Autodesk Fusion 360 part; units mm, degrees
note: some values were not read from the file. Set by a fixed rule: which face or edge a step refers to.
(part 3 of 5)
sketch "Sketch19" plane through (0, 5, 0) normal (0, 1, 0) x (-1, 0, 0)
  line L0 (-11.62, 44.17) -> (-67.5, 44.17) construction
  line L1 (-115.5, 44.17) -> (-115.5, -27.83) construction
  line L2 (-115.5, -27.83) -> (-120.5, -27.83) construction
  line L3 (-120.5, -27.83) -> (-120.5, -39.83) construction
  line L4 (-120.5, -39.83) -> (67.5, -39.83) construction
  line L5 (-72.5, 2.17) -> (-115.5, 2.17) construction
  circle A0 centre (-94, 2.17) radius 1.5
  circle A1 centre (-109, -33.83) radius 1.5
  circle A2 centre (-101.5, -33.83) radius 1.5
  circle A3 centre (-94, -33.83) radius 1.5
  circle A4 centre (-86.5, -33.83) radius 1.5
  circle A5 centre (-79, -33.83) radius 1.5
  circle A6 centre (-109, -21.83) radius 1.5
  circle A7 centre (-101.5, -21.83) radius 1.5
  circle A8 centre (-94, -21.83) radius 1.5
  circle A9 centre (-86.5, -21.83) radius 1.5
  circle A10 centre (-79, -21.83) radius 1.5
  circle A11 centre (-109, -9.83) radius 1.5
  circle A12 centre (-101.5, -9.83) radius 1.5
  circle A13 centre (-94, -9.83) radius 1.5
  circle A14 centre (-86.5, -9.83) radius 1.5
  circle A15 centre (-79, -9.83) radius 1.5
  circle A16 centre (-109, 2.17) radius 1.5
  circle A17 centre (-101.5, 2.17) radius 1.5
  circle A18 centre (-86.5, 2.17) radius 1.5
  circle A19 centre (-79, 2.17) radius 1.5
  circle A20 centre (-109, 14.17) radius 1.5
  circle A21 centre (-101.5, 14.17) radius 1.5
  circle A22 centre (-94, 14.17) radius 1.5
  circle A23 centre (-86.5, 14.17) radius 1.5
  circle A24 centre (-79, 14.17) radius 1.5
  circle A25 centre (-109, 26.17) radius 1.5
  circle A26 centre (-101.5, 26.17) radius 1.5
  circle A27 centre (-94, 26.17) radius 1.5
  circle A28 centre (-86.5, 26.17) radius 1.5
  circle A29 centre (-79, 26.17) radius 1.5
  circle A30 centre (-109, 38.17) radius 1.5
  circle A31 centre (-101.5, 38.17) radius 1.5
  circle A32 centre (-94, 38.17) radius 1.5
  circle A33 centre (-86.5, 38.17) radius 1.5
  circle A34 centre (-79, 38.17) radius 1.5
  line L6 (-79, -33.83) -> (-79, -21.83) construction
  line L7 (-79, -21.83) -> (-86.5, -21.83) construction
  line L8 (-86.5, -21.83) -> (-86.5, -33.83) construction
  line L9 (-86.5, -33.83) -> (-79, -33.83) construction
  line L10 (-79, -27.83) -> (-86.5, -27.83) construction
  line L11 (-82.75, -33.83) -> (-82.75, -21.83) construction
  circle A35 centre (-82.75, -27.83) radius 1.5
  circle A36 centre (-90.25, -27.83) radius 1.5
  circle A37 centre (-97.75, -27.83) radius 1.5
  circle A38 centre (-105.25, -27.83) radius 1.5
  circle A39 centre (-82.75, -15.83) radius 1.5
  circle A40 centre (-90.25, -15.83) radius 1.5
  circle A41 centre (-97.75, -15.83) radius 1.5
  circle A42 centre (-105.25, -15.83) radius 1.5
  circle A43 centre (-82.75, -3.83) radius 1.5
  circle A44 centre (-90.25, -3.83) radius 1.5
  circle A45 centre (-97.75, -3.83) radius 1.5
  circle A46 centre (-105.25, -3.83) radius 1.5
  circle A47 centre (-82.75, 8.17) radius 1.5
  circle A48 centre (-90.25, 8.17) radius 1.5
  circle A49 centre (-97.75, 8.17) radius 1.5
  circle A50 centre (-105.25, 8.17) radius 1.5
  circle A51 centre (-82.75, 20.17) radius 1.5
  circle A52 centre (-90.25, 20.17) radius 1.5
  circle A53 centre (-97.75, 20.17) radius 1.5
  circle A54 centre (-105.25, 20.17) radius 1.5
  circle A55 centre (-82.75, 32.17) radius 1.5
  circle A56 centre (-90.25, 32.17) radius 1.5
  circle A57 centre (-97.75, 32.17) radius 1.5
  circle A58 centre (-105.25, 32.17) radius 1.5
  circle A59 centre (-31.75, 6.0325) radius 1.5
  circle A60 centre (-31.75, -18.0975) radius 1.5
  circle A61 centre (-6.35, -18.0975) radius 1.5
  circle A62 centre (-6.35, 18.0975) radius 1.5
  circle A63 centre (19.05, 18.0975) radius 1.5
  circle A64 centre (6.35, -18.0975) radius 1.5
  circle A65 centre (31.75, 6.0325) radius 1.5
  circle A66 centre (44.45, -6.0325) radius 1.5
  circle A67 centre (38.1, 24.13) radius 1.5
  circle A68 centre (0, 24.13) radius 1.5
  circle A69 centre (-25.4, -24.13) radius 1.5
  circle A70 centre (-12.7, -24.13) radius 1.5
  circle A71 centre (12.7, 12.065) radius 1.5
  circle A72 centre (50.8, -24.13) radius 1.5
  circle A73 centre (-50.8, -24.13) radius 1.5
  circle A74 centre (12.7, -12.065) radius 1.5
  circle A75 centre (-25.4, -12.065) radius 1.5
  circle A76 centre (50.8, 12.065) radius 1.5
  circle A77 centre (-38.1, 0) radius 1.5
  circle A78 centre (-50.8, 24.13) radius 1.5
  circle A79 centre (-12.7, -12.065) radius 1.5
  circle A80 centre (-38.1, -12.065) radius 1.5
  circle A81 centre (-38.1, -24.13) radius 1.5
  circle A82 centre (25.4, 0) radius 1.5
  circle A83 centre (25.4, -24.13) radius 1.5
  circle A84 centre (12.7, -24.13) radius 1.5
  circle A85 centre (38.1, -12.065) radius 1.5
  circle A86 centre (-38.1, 24.13) radius 1.5
  circle A87 centre (0, 12.065) radius 1.5
  circle A88 centre (-25.4, 0) radius 1.5
  circle A89 centre (44.45, -18.0975) radius 1.5
  circle A90 centre (31.75, 18.0975) radius 1.5
  circle A91 centre (19.05, -18.0975) radius 1.5
  circle A92 centre (19.05, 6.0325) radius 1.5
  circle A93 centre (-6.35, 6.0325) radius 1.5
  circle A94 centre (-6.35, -6.0325) radius 1.5
  circle A95 centre (-31.75, -6.0325) radius 1.5
  circle A96 centre (-44.45, 6.0325) radius 1.5
  circle A97 centre (-31.75, 18.0975) radius 1.5
  circle A98 centre (-44.45, -18.0975) radius 1.5
  circle A99 centre (-19.05, -18.0975) radius 1.5
  circle A100 centre (-19.05, 18.0975) radius 1.5
  circle A101 centre (6.35, 18.0975) radius 1.5
  circle A102 centre (6.35, -6.0325) radius 1.5
  circle A103 centre (31.75, -6.0325) radius 1.5
  circle A104 centre (44.45, 6.0325) radius 1.5
  circle A105 centre (25.4, 24.13) radius 1.5
  circle A106 centre (38.1, 0) radius 1.5
  circle A107 centre (-50.8, -12.065) radius 1.5
  circle A108 centre (-25.4, 24.13) radius 1.5
  circle A109 centre (-38.1, 12.065) radius 1.5
  circle A110 centre (38.1, -24.13) radius 1.5
  circle A111 centre (-50.8, 0) radius 1.5
  circle A112 centre (50.8, -12.065) radius 1.5
  circle A113 centre (38.1, 12.065) radius 1.5
  circle A114 centre (-50.8, 12.065) radius 1.5
  circle A115 centre (0, -24.13) radius 1.5
  circle A116 centre (-12.7, 0) radius 1.5
  circle A117 centre (12.7, 24.13) radius 1.5
  circle A118 centre (25.4, 12.065) radius 1.5
  circle A119 centre (-25.4, 12.065) radius 1.5
  circle A120 centre (12.7, 0) radius 1.5
  circle A121 centre (-12.7, 24.13) radius 1.5
  circle A122 centre (25.4, -12.065) radius 1.5
  circle A123 centre (0, 0) radius 1.5
  circle A124 centre (50.8, 0) radius 1.5
  circle A125 centre (50.8, 24.13) radius 1.5
  circle A126 centre (0, -12.065) radius 1.5
  circle A127 centre (-12.7, 12.065) radius 1.5
  circle A128 centre (44.45, 18.0975) radius 1.5
  circle A129 centre (31.75, -18.0975) radius 1.5
  circle A130 centre (19.05, -6.0325) radius 1.5
  circle A131 centre (6.35, 6.0325) radius 1.5
  circle A132 centre (-19.05, 6.0325) radius 1.5
  circle A133 centre (-19.05, -6.0325) radius 1.5
  circle A134 centre (-44.45, -6.0325) radius 1.5
  circle A135 centre (-44.45, 18.0975) radius 1.5
  circle A136 centre (58.42, -31.75) radius 3.9
  circle A137 centre (58.42, 31.75) radius 3.9
  line L12 (67.5, 39.83) -> (-11.62, 39.83)
  line L13 (-11.62, 39.83) -> (-11.62, 44.17)
  line L14 (67.5, -39.83) -> (67.5, 39.83)
  circle A138 centre (-58.42, 31.75) radius 3.9
  circle A139 centre (-58.42, -31.75) radius 3.9
  line L15 (-67.5, 44.17) -> (-67.5, -22.83)
  line L16 (-67.5, -22.83) -> (-72.5, -22.83)
  line L17 (-72.5, -22.83) -> (-72.5, 44.17)
  line L18 (-72.5, 44.17) -> (-115.5, 44.17)
  line L19 (-94, 44.17) -> (-94, -39.83) construction
  line L20 (-72.5, 44.17) -> (-72.5, -39.83) construction
  dimension "d176" = 3
  dimension "d179" = 15
  dimension "d180" = 36
  dimension "d181" = 3
  dimension "d184" = -22.5
  dimension "d185" = 60
  constraint coincident L1 L5.end
  constraint perpendicular L1 L5
  constraint coincident A5.centre L6.start
  constraint coincident A10.centre L6.end
  constraint coincident A9.centre L7.end
  constraint coincident A4.centre L8.end
  constraint midpoint L6 L10.start
  constraint midpoint L8 L10.end
  constraint midpoint L9 L11.start
  constraint midpoint L7 L11.end
  constraint midpoint L10 A35.centre
  constraint midpoint L18 L19.start
  constraint coincident L4 L19.end
  constraint vertical L19
  constraint coincident L5 A0.centre
  constraint coincident A0.centre L19
  constraint coincident L17.end L18.start
  constraint coincident L4 L20.end
  constraint perpendicular L4 L20
  constraint midpoint L5.start L20
  measures "d176" diameter of A0
  measures "d181" diameter of A35
extrude "Extrude22" cut sketch "Sketch19" against normal up to surface (5 mm away) contours A0 | A1 | A2 | A3 | A4 | A5 | A6 | A7 | A8 | A9 | A10 | A11 | A12 | A13 | A14 | A15 | A16 | A17 | A18 | A19 | A20 | A21 | A22 | A23 | A24 | A25 | A26 | A27 | A28 | A29 | A30 | A31 | A32 | A33 | A34 | A35 | A36 | A37 | A38 | A39 | A40 | A41 | A42 | A43 | A44 | A45 | A46 | A47 | A48 | A49 | A50 | A51 | A52 | A53 | A54 | A55 | A56 | A57 | A58 bodies 1
fillet "Fillet2" [suppressed]
equation "d1 = 5 in + 8 mm"
equation "d2 = d1 / 2"
equation "d3 = 2.9 in + 6 mm"
equation "d4 = d3 / 2"
equation "d9 = d1 / 2 - 0.2 in - 4 mm"
equation "d10 = d9"
equation "d11 = d9"
equation "d12 = d9"
equation "d13 = d3 / 2 - 0.2 in - 3 mm"
equation "d14 = d13"
equation "d15 = d13"
equation "d16 = d13"
equation "d18 = d17"
equation "d19 = d17"
equation "d20 = d18"
equation "d21 = d17 + 4 mm"
equation "d22 = d21"
equation "d23 = d21"
equation "d24 = d21"
equation "d25 = 5 mm"
equation "d29 = d25 + 30 mm"
equation "d39 = d33 / 2"
equation "d40 = d39"
equation "d42 = d39"
equation "d43 = d121"
equation "d44 = d41"
equation "d46 = d39"
equation "d47 = d41"
equation "d48 = d39"
equation "d50 = d41"
equation "d60 = 2.8 in + 8 mm"
equation "d63 = 1.65 in + 8 mm - d29"
equation "d66 = d65"
equation "d67 = d65"
equation "d69 = -d59 + 3 mm"
equation "d80 = d79"
equation "d81 = d79"
equation "d82 = d79"
equation "d85 = 0.2 in + 1 mm"
equation "d86 = d85"
equation "d87 = d85"
equation "d88 = d85"
equation "d89 = d85"
equation "d91 = d85"
equation "d113 = d5"
equation "d114 = d8"
equation "d115 = d8"
equation "d116 = d33"
equation "d122 = d39"
equation "d131 = d85"
equation "d132 = d85"
equation "d133 = d79 + 3 mm"
equation "d134 = d133"
equation "d135 = d133"
equation "d136 = d133"
equation "d140 = d65"
equation "d171 = d168"
equation "d181 = d176"

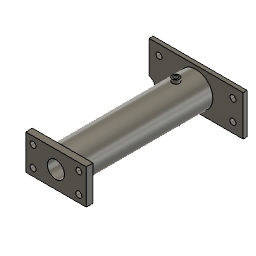
design "Measurement Tube Front Adapter"
Autodesk Fusion 360 part; units mm, degrees
sketch "Sketch1" plane through (0, 0, 0) normal (0, 0, 1) x (1, 0, 0)
  circle A0 centre (0, 0) radius 7
  circle A1 centre (0, 0) radius 12.5
  dimension "d1" = 25
  dimension "d2" = 14
  constraint coincident A0.centre A1.centre
  measures "d1" diameter of A1
  measures "d2" diameter of A0
extrude "Extrude1" add sketch "Sketch1" along normal blind 15 contours A0 | A1
sketch "Sketch2" plane through (0, 0, 15) normal (0, 0, 1) x (1, 0, 0)
  circle A0 centre (0, 0) radius 12.5
  circle A1 centre (0, 0) radius 6.375
  dimension "d5" = 12.75
  constraint concentric A0 A1
  measures "d5" diameter of A1
loft "Loft1" cut profiles "Sketch1", "Sketch2" section 1 contours A0 section 2 contours A1
extrude "Extrude2" add 1 faces at (10.4118, -0.621, 15) along direction (0, 0, 1) blind 92
sketch "Sketch17" plane through (0, 0, 107) normal (0, 0, 1) x (1, 0, 0)
  circle A0 centre (-17, -7.5) radius 2.25
  circle A1 centre (17, -7.5) radius 2.25
  circle A2 centre (0, 0) radius 6.375
  circle A3 centre (0, 0) radius 12.5
  line L0 (-22.5, 13) -> (22.5, 13)
  line L1 (22.5, 13) -> (22.5, -13)
  line L2 (22.5, -13) -> (-22.5, -13)
  line L3 (-22.5, -13) -> (-22.5, 13)
  line L4 (0, 0) -> (-22.5, 0) construction
  line L5 (0, 0) -> (22.5, 0) construction
  circle A4 centre (-17, 7.5) radius 2.25
  circle A5 centre (17, 7.5) radius 2.25
  point P0 (-12.5, 0)
  point P1 (12.5, 0)
  dimension "d112" = 4.5
  dimension "d113" = 4.5
  dimension "d147" = 10
  dimension "d148" = 10
  dimension "d149" = 7.5
  dimension "d150" = 13
  dimension "d151" = 17
  dimension "d152" = 17
  dimension "d153" = 7.5
  dimension "d154" = 17
  dimension "d155" = 7.5
  dimension "d156" = 4.5
  dimension "d157" = 4.5
  dimension "d158" = 17
  dimension "d159" = 7.5
  constraint horizontal L0
  constraint vertical L1
  constraint horizontal L2
  constraint vertical L3
  constraint coincident A2.centre A3.centre
  constraint midpoint L3 L4.end
  constraint midpoint L1 L5.end
  constraint horizontal L4
  constraint coincident A3 P0
  constraint coincident L4 P0
  constraint coincident L5 P1
  constraint coincident A3 P1
  measures "d112" diameter of A0
  measures "d113" diameter of A1
  measures "d147" distance of L4.end P0
  measures "d148" distance of L5.end P1
  measures "d149" distance of A0.centre L4
  measures "d150" distance of L2 L4
  measures "d151" horizontal distance of A0.centre A2.centre
  measures "d152" horizontal distance of A1.centre A2.centre
  measures "d153" distance of A1.centre L5
  measures "d154" horizontal distance of A2.centre A4.centre
  measures "d155" distance of L4 A4.centre
  measures "d156" diameter of A4
  measures "d157" diameter of A5
  measures "d158" horizontal distance of A2.centre A5.centre
  measures "d159" distance of L5 A5.centre
extrude "Extrude15" add sketch "Sketch17" against normal blind 5 contours A3 | L0 L1 L2 L3
sketch "Sketch18" plane through (0, 0, 0) normal (0, 0, -1) x (-1, 0, 0)
  circle A0 centre (-17, -7.5) radius 2.25
  circle A1 centre (17, -7.5) radius 2.25
  line L0 (-34.9564, 15) -> (34.9564, 15)
  line L1 (34.9564, 15) -> (34.9564, -15)
  line L2 (34.9564, -15) -> (-34.9564, -15)
  line L3 (-34.9564, -15) -> (-34.9564, 15)
  circle A2 centre (-27.4564, -7.5) radius 2.25
  circle A3 centre (0, 0) radius 7
  circle A4 centre (0, 0) radius 12.5
  line L4 (-22.5, -13) -> (22.5, -13)
  line L5 (22.5, -13) -> (22.5, 13)
  line L6 (22.5, 13) -> (-22.5, 13)
  line L7 (-22.5, 13) -> (-22.5, -13)
  circle A5 centre (0, 0) radius 12.5
  circle A6 centre (-17, 7.5) radius 2.25
  circle A7 centre (17, 7.5) radius 2.25
  circle A8 centre (-27.4564, 7.5) radius 2.25
  circle A9 centre (27.4564, 7.5) radius 2.25
  point P0 (0, -15)
  dimension "d122" = 4.5
  dimension "d124" = 7.5
  dimension "d125" = 7.5
  dimension "d160" = 34.9564
  dimension "d161" = 15
  dimension "d162" = 34.9564
  dimension "d163" = 15
  dimension "d164" = 7.5
  dimension "d165" = 7.5
  dimension "d166" = 4.5
  dimension "d167" = 7.5
  dimension "d168" = 7.5
  dimension "d169" = 4.5
  constraint horizontal L0
  constraint vertical L1
  constraint horizontal L2
  constraint vertical L3
  constraint midpoint L2 P0
  measures "d122" diameter of A2
  measures "d124" distance of L2 A2.centre
  measures "d125" distance of L3 A2.centre
  measures "d160" distance of A3.centre L3
  measures "d161" distance of A3.centre L2
  measures "d162" distance of L1.end P0
  measures "d163" distance of A3.centre L0
  measures "d164" distance of L0 A8.centre
  measures "d165" distance of L3 A8.centre
  measures "d166" diameter of A8
  measures "d167" distance of L1 A9.centre
  measures "d168" distance of L0 A9.centre
  measures "d169" diameter of A9
extrude "Extrude16" add sketch "Sketch18" against normal blind 3 contours A0 | A1 | L0 L1 L2 L3 | L4 L5 L6 L7 | A6 | A7
ref_plane "WorkPlane5" through (0, -7, 0) normal (0, 1, 0) x (0, 0, 1)
sketch "Sketch19" plane through (0, -7, 0) normal (0, 1, 0) x (1, 0, 0)
  line L0 (6.375, -15) -> (-6.375, -15)
  line L1 (0, -15) -> (0, -107) construction
  circle A0 centre (0, -18) radius 1.7
  circle A1 centre (0, -18) radius 2.7
  line L2 (6.375, -107) -> (-6.375, -107)
  dimension "d131" = 3.4
  dimension "d132" = 5.4
  dimension "d139" = 3
  constraint midpoint L0 L1.start
  constraint concentric A0 A1
  constraint coincident L1 A0.centre
  constraint midpoint L1.end L2
  measures "d131" diameter of A0
  measures "d132" diameter of A1
  measures "d139" distance of L0 A0.centre
extrude "Extrude17" add sketch "Sketch19" against normal blind 8
extrude "Extrude18" cut sketch "Sketch19" along normal blind 2 and the other way blind 8 contours A0
ref_plane "WorkPlane7" through (0, 7, 0) normal (0, 1, 0) x (0, 0, 1)
sketch "Sketch22" plane through (0, 7, 0) normal (0, 1, 0) x (1, 0, 0)
  circle A0 centre (0, -18) radius 1.7
  circle A1 centre (0, -18) radius 2.7
  point P0 (0, -18)
  dimension "d171" = 3.4
  dimension "d172" = 5.4
  constraint coincident P0 A0.centre
  measures "d171" diameter of A0
  measures "d172" diameter of A1
extrude "Extrude21" add sketch "Sketch22" along normal blind 8
extrude "Extrude22" cut sketch "Sketch22" along normal blind 8 and the other way blind 2 contours A0
sketch "Sketch23" plane through (0, 0, 0) normal (0, 0, -1) x (-1, 0, 0)
  line L0 (-34.9564, -15) -> (34.9564, -15)
  line L1 (34.9564, -15) -> (34.9564, 15)
  line L2 (34.9564, 15) -> (-34.9564, 15)
  line L3 (-34.9564, 15) -> (-34.9564, -15)
  circle A0 centre (-27.4564, 7.5) radius 2.25
  circle A1 centre (-27.4564, -7.5) radius 2.25
  circle A2 centre (27.4564, 7.5) radius 2.25
  circle A3 centre (0, 0) radius 7
  line L4 (34.9564, -15) -> (30.1724, -15)
  line L5 (34.9564, -9.125) -> (34.9564, -15)
  arc A4 (34.9564, -9.125) -> (30.1724, -15) centre (36.8966, -15.5902) ccw
  dimension "d181" = 4.784
  dimension "d182" = 5.875
  dimension "d183" = 6.75
  constraint horizontal L4
  constraint vertical L5
  constraint coincident L0.end L1.start
  measures "d181" distance of L0.end L4.end
  measures "d182" distance of L0.end L5.start
  measures "d183" radius of A4
extrude "Extrude23" cut sketch "Sketch23" against normal up to surface (3 mm away) contours L0 L1 L4 L5 A4
equation "d110 = 15 mm"
equation "d113 = d112"
equation "d116 = d110 / 2"
equation "d125 = d124"
equation "d130 = -d2 / 2"
equation "d132 = d131 + 2 mm"
equation "d148 = d147"
equation "d152 = d151"
equation "d153 = d149"
equation "d154 = d151"
equation "d155 = d149"
equation "d156 = d112"
equation "d157 = d112"
equation "d158 = d151"
equation "d159 = d149"
equation "d162 = d160"
equation "d163 = d161"
equation "d164 = d124"
equation "d165 = d124"
equation "d166 = d122"
equation "d167 = d124"
equation "d168 = d124"
equation "d169 = d122"
equation "d170 = ( d2 / 2 mm ) * 1 mm"
equation "d172 = d171 + 2 mm"
equation "d64 = d67"
equation "d67 = 40.00 mm"
equation "d70 = d67"
equation "d82 = -d67"
equation "d96 = d26 / 2"
equation "d97 = d16 / 2"
equation "d101 = -d29"
equation "d105 = -d29"
equation "d114 = 17 mm"
equation "d115 = d114"
equation "d117 = d116"
equation "d126 = d124"
equation "d127 = d124"

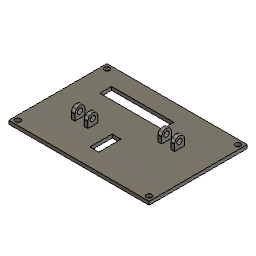
design "RPi Board Cover"
Autodesk Fusion 360 part; units mm, degrees
sketch "Sketch2" plane through (0, 0, 0) normal (0, 1, 0) x (1, 0, 0)
  line L0 (-60, 42) -> (60, 42)
  line L1 (60, 42) -> (60, -42)
  line L2 (60, -42) -> (-60, -42)
  line L3 (-60, -42) -> (-60, 42)
  line L4 (-41, 27) -> (12, 27)
  line L5 (12, 27) -> (12, 17)
  line L6 (12, 17) -> (-41, 17)
  line L7 (-41, 17) -> (-41, 27)
  line L8 (-5.5, -8) -> (2, -8)
  line L9 (2, -8) -> (2, -27)
  line L10 (2, -27) -> (-5.5, -27)
  line L11 (-5.5, -27) -> (-5.5, -8)
  circle A0 centre (-56, 38) radius 2.25
  circle A1 centre (56, 38) radius 2.25
  circle A2 centre (56, -38) radius 2.25
  circle A3 centre (-56, -38) radius 2.25
  line L12 (-56, 38) -> (-56, -38) construction
  line L13 (-56, -38) -> (56, -38) construction
  line L14 (56, -38) -> (56, 38) construction
  line L15 (56, 38) -> (-56, 38) construction
  dimension "d21" = 120
  dimension "d22" = 60
  dimension "d23" = 84
  dimension "d24" = 42
  dimension "d25" = 19
  dimension "d26" = 15
  dimension "d27" = 10
  dimension "d28" = 53
  dimension "d29" = 15
  dimension "d30" = 7.5
  dimension "d31" = 54.5
  dimension "d32" = 19
  dimension "d40" = 4
  dimension "d41" = 4
  dimension "d42" = 4
  dimension "d43" = 4
  dimension "d44" = 4.5
  constraint horizontal L0
  constraint vertical L1
  constraint horizontal L2
  constraint vertical L3
  constraint horizontal L4
  constraint vertical L5
  constraint horizontal L6
  constraint vertical L7
  constraint horizontal L8
  constraint vertical L9
  constraint horizontal L10
  constraint vertical L11
  constraint equal A0 A1
  constraint equal A0 A2
  constraint equal A0 A3
  constraint coincident A0.centre L12.start
  constraint coincident A3.centre L12.end
  constraint coincident A2.centre L13.end
  constraint horizontal L13
  constraint coincident A1.centre L14.end
  constraint parallel L13 L15
  constraint perpendicular L12 L15
  constraint perpendicular L14 L15
  measures "d21" distance of L0.start L0.end
  measures "d22" distance of origin L1
  measures "d23" distance of L0.start L2.end
  measures "d24" distance of origin L0
  measures "d25" distance of L3 L7
  measures "d26" distance of L0 L4
  measures "d27" distance of L4.start L6.end
  measures "d28" distance of L4.start L4.end
  measures "d29" distance of L2 L10
  measures "d30" distance of L8.start L8.end
  measures "d31" distance of L3 L11
  measures "d32" distance of L8.start L10.end
  measures "d40" distance of L0 L15
  measures "d41" distance of L2 L13
  measures "d42" distance of L3 L12
  measures "d43" distance of L1 L14
  measures "d44" diameter of A0
extrude "Extrude1" add sketch "Sketch2" along normal blind 3
ref_plane "WorkPlane1" through (-20, 0, 0) normal (1, 0, 0) x (0, 1, 0)
sketch "Sketch6" plane through (-20, 0, 0) normal (1, 0, 0) x (0, 0, -1)
  circle A0 centre (9.9499, 8.25) radius 4.25
  line L0 (5.6999, 8.25) -> (9.9499, 8.25) construction
  line L1 (9.9499, 8.25) -> (14.1999, 8.25) construction
  circle A1 centre (9.9499, 8.25) radius 2.25
  line L2 (5.6999, 8.25) -> (5.6999, 3)
  line L3 (14.1999, 8.25) -> (14.1999, 3)
  line L4 (-42, 3) -> (42, 3)
  line L5 (9.9499, 8.25) -> (9.9499, 4) construction
  point P0 (0, 3)
  dimension "d33" = 4.5
  dimension "d34" = 8.5
  dimension "d45" = 10
  dimension "d54" = 1
  constraint coincident A0 L0.start
  constraint coincident A0.centre L0.end
  constraint horizontal L0
  constraint coincident A0 L1.end
  constraint parallel L0 L1
  constraint tangent A0 L2
  constraint perpendicular L1 L3
  constraint coincident L2.end L4
  constraint coincident L3.end L4
  constraint coincident L1.end L3.start
  constraint coincident A0 L5.end
  constraint perpendicular L1 L5
  constraint midpoint L4 P0
  measures "d33" diameter of A1
  measures "d34" diameter of A0
  measures "d45" distance of L5.end P0
  measures "d54" distance of L4 L5.end
extrude "Extrude5" add sketch "Sketch6" against normal blind 14
ref_plane "WorkPlane3" through (-27, 0, 0) normal (1, 0, 0) x (0, 1, 0)
sketch "Sketch7" plane through (-27, 0, 0) normal (1, 0, 0) x (0, 0, -1)
  circle A0 centre (9.9499, 8.25) radius 2.25
  arc A1 (14.1999, 8.25) -> (5.6999, 8.25) centre (9.9499, 8.25) ccw
  line L0 (5.6999, 8.25) -> (5.6999, 3)
  line L1 (5.6999, 3) -> (14.1999, 3)
  line L2 (14.1999, 3) -> (14.1999, 8.25)
extrude "Extrude6" cut sketch "Sketch7" along normal mid plane 8
pattern_linear "R-Pattern1" count 2 spacing 20 along (0, 0, 1) count 2 spacing 54 along (1, 0, 0) of "Extrude5", "Extrude6"
extrude "Extrude7" cut 1 faces at (-34, 4.0021, -10.0059) along direction (1, 0, 0) up to surface (14 mm away)
extrude "Extrude8" cut 1 faces at (20, 4.0021, 9.9941) along direction (1, 0, 0) up to surface (14 mm away)
equation "d3 = -20.00 mm"
equation "d22 = d21 / 2"
equation "d24 = d23 / 2"
equation "d34 = d33 + 4 mm"
equation "d35 = -14.00 mm"
equation "d37 = d3 + ( d35 / 2 mm ) * 1 mm"
equation "d41 = d40"
equation "d42 = d40"
equation "d43 = d42"
equation "d48 = 2 * d45"
equation "d49 = d37 * -2"

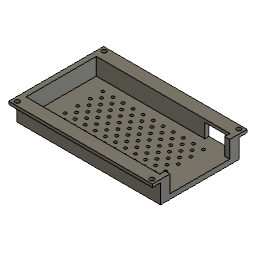
design "Portable Battery Case"
Autodesk Fusion 360 part; units mm, degrees
sketch "Sketch1" plane through (0, 0, 0) normal (0, 1, 0) x (1, 0, 0)
  line L0 (-66.4, 34.9) -> (66.4, 34.9)
  line L1 (66.4, 34.9) -> (66.4, -34.9)
  line L2 (66.4, -34.9) -> (-66.4, -34.9)
  line L3 (-66.4, -34.9) -> (-66.4, 34.9)
  line L4 (-71.4, -39.15) -> (71.4, -39.15)
  line L5 (71.4, 39.15) -> (71.4, -39.15)
  line L6 (0, 0) -> (-71.6, 0) construction
  line L7 (-71.4, 39.15) -> (71.4, 39.15)
  line L8 (-71.4, 39.15) -> (-71.4, -39.15)
  dimension "d1" = 69.8
  dimension "d2" = 132.8
  dimension "d3" = 66.4
  dimension "d4" = 34.9
  dimension "d40" = 4.25
  dimension "d46" = 4.25
  dimension "d47" = 5
  dimension "d63" = 5
  constraint horizontal L0
  constraint vertical L1
  constraint horizontal L2
  constraint vertical L3
  constraint coincident L6.start origin
  constraint horizontal L6
  constraint perpendicular L5 L7
  constraint perpendicular L4 L5
  constraint perpendicular L7 L8
  measures "d1" distance of L0.start L2.end
  measures "d2" distance of L0.start L0.end
  measures "d3" distance of L6.start L3
  measures "d4" distance of L6.start L0
  measures "d40" distance of L2 L4
  measures "d46" distance of L0 L7
  measures "d47" distance of L1 L5
  measures "d63" distance of L3 L8
extrude "Extrude1" add sketch "Sketch1" along normal blind 5 contours L0 L1 L2 L3
extrude "Extrude2" add sketch "Sketch1" along normal blind 22.018
sketch "Sketch3" plane through (0, 22.018, 0) normal (0, 1, 0) x (-1, 0, 0)
  line L0 (-66.4, 34.9) -> (66.4, 34.9)
  line L1 (66.4, 34.9) -> (66.4, -34.9)
  line L2 (66.4, -34.9) -> (-66.4, -34.9)
  line L3 (-66.4, -34.9) -> (-66.4, 34.9)
  line L4 (62.4, -47.15) -> (-71.4, -47.15)
  line L5 (-71.4, -47.15) -> (-71.4, 47.15)
  line L6 (-71.4, 47.15) -> (71.4, 47.15)
  circle A0 centre (66.9, -43.15) radius 2.25
  circle A1 centre (-66.9, -43.15) radius 2.25
  circle A2 centre (-66.9, 43.15) radius 2.25
  circle A3 centre (66.9, 43.15) radius 2.25
  line L7 (71.4, 39.15) -> (-71.4, 39.15)
  line L8 (-71.4, 39.15) -> (-71.4, -39.15)
  line L9 (-71.4, -39.15) -> (71.4, -39.15)
  line L10 (62.4, -47.15) -> (71.4, -47.15)
  line L11 (71.4, 39.15) -> (71.4, 47.15)
  line L12 (71.4, -39.15) -> (71.4, 39.15)
  line L13 (71.4, -47.15) -> (71.4, -39.15)
  point P0 (-71.4, 0)
  point P1 (71.4, 39.15)
  dimension "d23" = 4.5
  dimension "d24" = 4
  dimension "d25" = 4.5
  dimension "d26" = 4.5
  dimension "d27" = 4
  dimension "d29" = 4.5
  dimension "d30" = 4.5
  dimension "d31" = 4
  dimension "d32" = 4.5
  dimension "d50" = 9
  dimension "d51" = 4.5
  dimension "d52" = 4
  dimension "d64" = 8
  dimension "d65" = 8
  dimension "d66" = 4.5
  constraint horizontal L4
  constraint vertical L5
  constraint horizontal L6
  constraint midpoint L5 P0
  constraint coincident L8.end L5
  constraint coincident P1 L7.start
  constraint perpendicular L6 L11
  constraint perpendicular L9 L13
  constraint coincident L9.end L12.start
  constraint perpendicular L10 L13
  measures "d23" diameter of A0
  measures "d24" distance of L4 A1.centre
  measures "d25" distance of L5 A1.centre
  measures "d26" diameter of A1
  measures "d27" distance of L6 A3.centre
  measures "d29" diameter of A3
  measures "d30" distance of L5 A2.centre
  measures "d31" distance of L6 A2.centre
  measures "d32" diameter of A2
  measures "d50" distance of L4.start L10.end
  measures "d51" distance of A3.centre L11
  measures "d52" distance of A0.centre L10
  measures "d64" distance of L6 L7
  measures "d65" distance of L10.end L9.end
  measures "d66" distance of A0.centre L13
extrude "Extrude4" add sketch "Sketch3" against normal blind 3 contours L4 L5 L9 L10 L13 | L5 L6 L7 L11
sketch "Sketch2" plane through (71.4, 0, 0) normal (1, 0, 0) x (0, 0, -1)
  line L0 (39.65, 0) -> (39.65, 18.75)
  line L1 (-34.65, 5) -> (34.65, 5)
  line L2 (34.65, 5) -> (-34.65, 5)
  line L3 (-29.65, 22.018) -> (29.65, 22.018)
  line L4 (29.65, 22.018) -> (29.65, 5)
  line L5 (29.65, 5) -> (-29.65, 5)
  line L6 (-29.65, 5) -> (-29.65, 22.018)
  line L7 (-39.15, 0) -> (39.15, 0)
  line L8 (39.15, 19.018) -> (47.15, 19.018)
  line L9 (47.15, 19.018) -> (47.15, 22.018)
  line L10 (47.15, 22.018) -> (-47.15, 22.018)
  line L11 (-47.15, 22.018) -> (-47.15, 19.018)
  line L12 (-47.15, 19.018) -> (-39.15, 19.018)
  line L13 (-39.15, 19.018) -> (-39.15, 0)
  line L14 (39.15, 0) -> (39.15, 19.018)
  point P0 (0, 22.018)
  dimension "d13" = 5
  dimension "d14" = 5
  constraint horizontal L3
  constraint vertical L4
  constraint horizontal L5
  constraint vertical L6
  constraint coincident L2 L4.end
  constraint midpoint L3 P0
  constraint coincident L10 P0
  measures "d13" distance of L1.start L6
  measures "d14" distance of L1.end L4
extrude "Extrude3" cut sketch "Sketch2" against normal up to surface (5 mm away) contours L1 L2 L3 L4 L5 L6 L10
sketch "Sketch6" plane through (0, 5, 0) normal (0, 1, 0) x (-1, 0, 0)
  line L0 (66.4, 34.9) -> (-66.4, 34.9)
  line L1 (-66.4, 34.9) -> (-66.4, 29.65)
  line L2 (-66.4, 29.65) -> (-71.4, 29.65)
  line L3 (-71.4, 29.65) -> (-71.4, -29.65)
  line L4 (-71.4, -29.65) -> (-66.4, -29.65)
  line L5 (-66.4, -29.65) -> (-66.4, -34.9)
  line L6 (-66.4, -34.9) -> (66.4, -34.9)
  line L7 (66.4, -34.9) -> (66.4, 34.9)
  circle A0 centre (0, 0) radius 1.5
  circle A1 centre (-50, -25) radius 1.5
  circle A2 centre (-40, -25) radius 1.5
  circle A3 centre (-30, -25) radius 1.5
  circle A4 centre (-20, -25) radius 1.5
  circle A5 centre (-10, -25) radius 1.5
  circle A6 centre (0, -25) radius 1.5
  circle A7 centre (10, -25) radius 1.5
  circle A8 centre (20, -25) radius 1.5
  circle A9 centre (30, -25) radius 1.5
  circle A10 centre (40, -25) radius 1.5
  circle A11 centre (50, -25) radius 1.5
  circle A12 centre (-50, -12.5) radius 1.5
  circle A13 centre (-40, -12.5) radius 1.5
  circle A14 centre (-30, -12.5) radius 1.5
  circle A15 centre (-20, -12.5) radius 1.5
  circle A16 centre (-10, -12.5) radius 1.5
  circle A17 centre (0, -12.5) radius 1.5
  circle A18 centre (10, -12.5) radius 1.5
  circle A19 centre (20, -12.5) radius 1.5
  circle A20 centre (30, -12.5) radius 1.5
  circle A21 centre (40, -12.5) radius 1.5
  circle A22 centre (50, -12.5) radius 1.5
  circle A23 centre (-50, 0) radius 1.5
  circle A24 centre (-40, 0) radius 1.5
  circle A25 centre (-30, 0) radius 1.5
  circle A26 centre (-20, 0) radius 1.5
  circle A27 centre (-10, 0) radius 1.5
  circle A28 centre (10, 0) radius 1.5
  circle A29 centre (20, 0) radius 1.5
  circle A30 centre (30, 0) radius 1.5
  circle A31 centre (40, 0) radius 1.5
  circle A32 centre (50, 0) radius 1.5
  circle A33 centre (-50, 12.5) radius 1.5
  circle A34 centre (-40, 12.5) radius 1.5
  circle A35 centre (-30, 12.5) radius 1.5
  circle A36 centre (-20, 12.5) radius 1.5
  circle A37 centre (-10, 12.5) radius 1.5
  circle A38 centre (0, 12.5) radius 1.5
  circle A39 centre (10, 12.5) radius 1.5
  circle A40 centre (20, 12.5) radius 1.5
  circle A41 centre (30, 12.5) radius 1.5
  circle A42 centre (40, 12.5) radius 1.5
  circle A43 centre (50, 12.5) radius 1.5
  circle A44 centre (-50, 25) radius 1.5
  circle A45 centre (-40, 25) radius 1.5
  circle A46 centre (-30, 25) radius 1.5
  circle A47 centre (-20, 25) radius 1.5
  circle A48 centre (-10, 25) radius 1.5
  circle A49 centre (0, 25) radius 1.5
  circle A50 centre (10, 25) radius 1.5
  circle A51 centre (20, 25) radius 1.5
  circle A52 centre (30, 25) radius 1.5
  circle A53 centre (40, 25) radius 1.5
  circle A54 centre (50, 25) radius 1.5
  line L8 (50, -25) -> (40, -25) construction
  line L9 (40, -25) -> (40, -12.5) construction
  line L10 (40, -12.5) -> (50, -12.5) construction
  line L11 (50, -12.5) -> (50, -25) construction
  line L12 (50, -18.75) -> (40, -18.75) construction
  line L13 (45, -25) -> (45, -12.5) construction
  circle A55 centre (45, -18.75) radius 1.5
  circle A56 centre (35, -18.75) radius 1.5
  circle A57 centre (25, -18.75) radius 1.5
  circle A58 centre (15, -18.75) radius 1.5
  circle A59 centre (5, -18.75) radius 1.5
  circle A60 centre (-5, -18.75) radius 1.5
  circle A61 centre (-15, -18.75) radius 1.5
  circle A62 centre (-25, -18.75) radius 1.5
  circle A63 centre (-35, -18.75) radius 1.5
  circle A64 centre (-45, -18.75) radius 1.5
  circle A65 centre (45, -6.25) radius 1.5
  circle A66 centre (35, -6.25) radius 1.5
  circle A67 centre (25, -6.25) radius 1.5
  circle A68 centre (15, -6.25) radius 1.5
  circle A69 centre (5, -6.25) radius 1.5
  circle A70 centre (-5, -6.25) radius 1.5
  circle A71 centre (-15, -6.25) radius 1.5
  circle A72 centre (-25, -6.25) radius 1.5
  circle A73 centre (-35, -6.25) radius 1.5
  circle A74 centre (-45, -6.25) radius 1.5
  circle A75 centre (45, 6.25) radius 1.5
  circle A76 centre (35, 6.25) radius 1.5
  circle A77 centre (25, 6.25) radius 1.5
  circle A78 centre (15, 6.25) radius 1.5
  circle A79 centre (5, 6.25) radius 1.5
  circle A80 centre (-5, 6.25) radius 1.5
  circle A81 centre (-15, 6.25) radius 1.5
  circle A82 centre (-25, 6.25) radius 1.5
  circle A83 centre (-35, 6.25) radius 1.5
  circle A84 centre (-45, 6.25) radius 1.5
  circle A85 centre (45, 18.75) radius 1.5
  circle A86 centre (35, 18.75) radius 1.5
  circle A87 centre (25, 18.75) radius 1.5
  circle A88 centre (15, 18.75) radius 1.5
  circle A89 centre (5, 18.75) radius 1.5
  circle A90 centre (-5, 18.75) radius 1.5
  circle A91 centre (-15, 18.75) radius 1.5
  circle A92 centre (-25, 18.75) radius 1.5
  circle A93 centre (-35, 18.75) radius 1.5
  circle A94 centre (-45, 18.75) radius 1.5
  dimension "d67" = 3
  dimension "d70" = 50
  dimension "d71" = 25
  dimension "d72" = 3
  dimension "d75" = -90
  dimension "d76" = 37.5
  constraint coincident A0.centre origin
  constraint horizontal L8
  constraint vertical L9
  constraint horizontal L10
  constraint vertical L11
  constraint coincident A21.centre L9.end
  constraint coincident A11.centre L8.start
  constraint midpoint L11 L12.start
  constraint midpoint L9 L12.end
  constraint midpoint L8 L13.start
  constraint midpoint L10 L13.end
  constraint midpoint L13 A55.centre
  measures "d67" diameter of A0
  measures "d72" diameter of A55
extrude "Extrude7" cut sketch "Sketch6" against normal up to surface (5 mm away) contours A0 | A1 | A2 | A3 | A4 | A5 | A6 | A7 | A8 | A9 | A10 | A11 | A12 | A13 | A14 | A15 | A16 | A17 | A18 | A19 | A20 | A21 | A22 | A23 | A24 | A25 | A26 | A27 | A28 | A29 | A30 | A31 | A32 | A33 | A34 | A35 | A36 | A37 | A38 | A39 | A40 | A41 | A42 | A43 | A44 | A45 | A46 | A47 | A48 | A49 | A50 | A51 | A52 | A53 | A54 | A55 | A56 | A57 | A58 | A59 | A60 | A61 | A62 | A63 | A64 | A65 | A66 | A67 | A68 | A69 | A70 | A71 | A72 | A73 | A74 | A75 | A76 | A77 | A78 | A79 | A80 | A81 | A82 | A83 | A84 | A85 | A86 | A87 | A88 | A89 | A90 | A91 | A92 | A93 | A94
sketch "Sketch7" plane through (0, 0, -39.15) normal (0, 0, -1) x (-1, 0, 0)
  line L0 (71.4, 19.018) -> (-71.4, 19.018)
  line L1 (-71.4, 19.018) -> (-71.4, 0)
  line L2 (-71.4, 0) -> (71.4, 0)
  line L3 (71.4, 0) -> (71.4, 19.018)
  line L4 (66.4, 5) -> (-66.4, 5)
  line L5 (-66.4, 5) -> (-66.4, 22.018)
  line L6 (-66.4, 22.018) -> (66.4, 22.018)
  line L7 (66.4, 22.018) -> (66.4, 5)
  line L8 (-61.4, 5) -> (-41.4, 5)
  line L9 (-41.4, 5) -> (-41.4, 19.018)
  line L10 (-41.4, 19.018) -> (-61.4, 19.018)
  line L11 (-61.4, 19.018) -> (-61.4, 5)
  dimension "d83" = 5
  dimension "d84" = 20
  constraint horizontal L8
  constraint vertical L9
  constraint horizontal L10
  constraint vertical L11
  constraint coincident L4 L8.start
  constraint coincident L0 L10.end
  measures "d83" distance of L5 L11
  measures "d84" distance of L8.start L8.end
extrude "Extrude8" cut sketch "Sketch7" against normal up to surface (4.25 mm away) contours L0 L4 L8 L9 L10 L11
fillet "Fillet1" [suppressed]
equation "d3 = d2 / 2"
equation "d4 = d1 / 2"
equation "d9 = 5 mm"
equation "d11 = d9 + 0.67 in"
equation "d14 = d13"
equation "d24 = d27"
equation "d25 = d30"
equation "d26 = d23"
equation "d27 = d64 / 2"
equation "d29 = d23"
equation "d31 = d27"
equation "d32 = d23"
equation "d46 = d40"
equation "d51 = d30"
equation "d52 = d27"
equation "d63 = d47"
equation "d65 = d64"
equation "d66 = d30"
equation "d72 = d67"

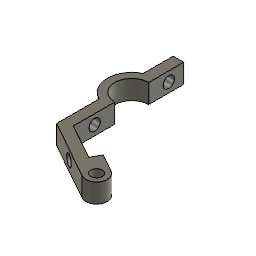
design "Trumpet Clamp 1 Main"
Autodesk Fusion 360 part; units mm, degrees
sketch "Sketch1" plane through (0, 0, 0) normal (0, 1, 0) x (1, 0, 0)
  circle A0 centre (0, 0) radius 6.755
  circle A1 centre (0, 0) radius 9.755
  line L0 (0, 0) -> (-9.755, 0) construction
  line L1 (0, 0) -> (9.755, 0) construction
  line L2 (-4.25, -25.7687) -> (18.9274, -38.7154)
  line L3 (4.25, -20.7805) -> (23.0726, -31.2946)
  circle A2 centre (21, -35.005) radius 4.25
  line L4 (21, -35.005) -> (18.9274, -38.7154) construction
  line L5 (21, -35.005) -> (23.0726, -31.2946) construction
  circle A3 centre (21, -35.005) radius 2.25
  line L6 (-4.25, -25.7687) -> (-4.25, -8.7805)
  line L7 (4.25, -20.7805) -> (4.25, -8.7805)
  line L8 (0, 0) -> (0, -20.7805) construction
  line L9 (4.25, -20.7805) -> (-4.25, -20.7805) construction
  line L10 (-4.25, 8.7805) -> (-4.25, 20.7805)
  line L11 (-4.25, 20.7805) -> (4.25, 20.7805)
  line L12 (4.25, 20.7805) -> (4.25, 8.7805)
  line L13 (-4.25, 8.7805) -> (-4.25, -8.7805) construction
  line L14 (4.25, -8.7805) -> (4.25, 8.7805) construction
  line L15 (21, -35.005) -> (21, -39.255) construction
  point P0 (0, -9.755)
  dimension "d1" = 13.51
  dimension "d3" = 4.5
  dimension "d4" = 8.5
  dimension "d5" = 21
  dimension "d19" = 8.5
  dimension "d22" = 19.51
  dimension "d27" = 12
  dimension "d28" = 12
  dimension "d32" = 29.5
  constraint coincident A0.centre A1.centre
  constraint concentric A0 A1
  constraint coincident A1 L0.end
  constraint horizontal L0
  constraint coincident A1 L1.end
  constraint parallel L0 L1
  constraint coincident A2.centre L4.start
  constraint coincident A2 L2.end
  constraint coincident A2 L3.end
  constraint parallel L4 L5
  constraint coincident L2.end L4.end
  constraint coincident L3.end L5.end
  constraint coincident A1 L6.end
  constraint coincident A1 L7.end
  constraint parallel L2 L3
  constraint vertical L6
  constraint vertical L7
  constraint vertical L8
  constraint tangent L3 A2
  constraint coincident L6 L9.end
  constraint perpendicular L6 L9
  constraint midpoint L8.end L9
  constraint coincident A1 L10.start
  constraint vertical L10
  constraint perpendicular L10 L11
  constraint coincident A1 L12.end
  constraint perpendicular L11 L12
  constraint vertical L13
  constraint vertical L14
  constraint coincident A2 L15.end
  constraint vertical L15
  constraint coincident A1 P0
  constraint coincident L8 P0
  measures "d1" diameter of A0
  measures "d3" diameter of A3
  measures "d4" diameter of A2
  measures "d5" horizontal distance of A0.centre A2.centre
  measures "d19" distance of L6 L7
  measures "d22" diameter of A1
  measures "d27" distance of L3.start L7.end
  measures "d28" distance of L11.end L12.end
  measures "d32" vertical distance of L15.end P0
extrude "Extrude1" add sketch "Sketch1" along normal blind 7.7
sketch "Sketch2" plane through (-7.8365, 0, 14.0291) normal (0.487666, 0, -0.87303) x (-0.87303, 0, -0.487666)
  line L0 (-35.4044, 0) -> (-13.8443, 0)
  line L1 (-13.8443, 0) -> (-13.8443, 7.7)
  line L2 (-13.8443, 7.7) -> (-35.4044, 7.7)
  line L3 (-35.4044, 7.7) -> (-35.4044, 0)
  line L4 (-13.8443, 3.85) -> (-35.4044, 3.85) construction
  circle A0 centre (-21.8443, 3.85) radius 2.25
  dimension "d29" = 8
  dimension "d30" = 4.5
  constraint midpoint L1 L4.start
  constraint midpoint L3 L4.end
  constraint coincident L4 A0.centre
  measures "d29" distance of L4.start A0.centre
  measures "d30" diameter of A0
extrude "Extrude2" cut sketch "Sketch2" against normal up to surface (8.5 mm away) contours A0
sketch "Sketch3" plane through (4.25, 0, 0) normal (1, 0, 0) x (0, 0, -1)
  line L0 (-20.7805, 0) -> (-8.7805, 0)
  line L1 (-8.7805, 0) -> (-8.7805, 7.7)
  line L2 (-8.7805, 7.7) -> (-20.7805, 7.7)
  line L3 (-20.7805, 7.7) -> (-20.7805, 0)
  line L4 (-8.7805, 3.85) -> (-20.7805, 3.85) construction
  circle A0 centre (-14.7805, 3.85) radius 2.25
  line L5 (8.7805, 0) -> (20.7805, 0)
  line L6 (20.7805, 0) -> (20.7805, 7.7)
  line L7 (20.7805, 7.7) -> (8.7805, 7.7)
  line L8 (8.7805, 7.7) -> (8.7805, 0)
  line L9 (8.7805, 3.85) -> (20.7805, 3.85) construction
  circle A1 centre (14.7805, 3.85) radius 2.25
  dimension "d16" = 4.5
  constraint midpoint L1 L4.start
  constraint midpoint L3 L4.end
  constraint midpoint L4 A0.centre
  constraint midpoint L8 L9.start
  constraint midpoint L6 L9.end
  constraint midpoint L9 A1.centre
  constraint equal A0 A1
  measures "d16" diameter of A0
extrude "Extrude3" cut sketch "Sketch3" against normal up to surface (8.5 mm away) contours A0 | A1
sketch "Sketch4" plane through (0, 0, 0) normal (1, 0, 0) x (0, 0, -1)
  line L0 (-20.7805, 0) -> (-8.7805, 0) construction
  line L1 (-8.7805, 0) -> (-8.7805, 7.7) construction
  line L2 (-8.7805, 7.7) -> (-20.7805, 7.7) construction
  line L3 (-20.7805, 7.7) -> (-20.7805, 0) construction
  line L4 (8.7805, 0) -> (-8.7805, 0) construction
  line L5 (-8.7805, 0) -> (-8.7805, 7.7) construction
  line L6 (8.7805, 7.7) -> (-8.7805, 7.7) construction
  line L7 (-8.7805, 7.7) -> (-8.7805, 0) construction
  line L8 (-8.7805, 0) -> (-25.7687, 0) construction
  line L9 (-25.7687, 0) -> (-25.7687, 7.7) construction
  line L10 (-25.7687, 7.7) -> (-8.7805, 7.7) construction
  line L11 (-8.7805, 7.7) -> (-8.7805, 0) construction
  line L12 (8.7805, 0) -> (-23.2746, 0)
  line L13 (-23.2746, 0) -> (-23.2746, 7.7)
  line L14 (-23.2746, 7.7) -> (8.7805, 7.7)
  line L15 (8.7805, 7.7) -> (8.7805, 0)
  line L16 (-25.7687, 7.7) -> (-20.7805, 7.7) construction
  line L17 (8.7805, 7.7) -> (8.7805, 0)
  line L18 (8.7805, 0) -> (-8.7805, 0)
  line L19 (8.7805, 0) -> (8.7805, 7.7)
  line L20 (8.7805, 7.7) -> (-8.7805, 7.7)
  circle A0 centre (14.7805, 3.85) radius 2.25
  line L21 (8.7805, 0) -> (20.7805, 0)
  line L22 (20.7805, 0) -> (20.7805, 7.7)
  line L23 (20.7805, 7.7) -> (8.7805, 7.7)
  line L24 (8.7805, 7.7) -> (8.7805, 0)
  circle A1 centre (-14.7805, 3.85) radius 2.25
  circle A2 centre (-14.7805, 3.85) radius 2.25
  constraint horizontal L12
  constraint vertical L13
  constraint horizontal L14
  constraint vertical L15
  constraint coincident L10 L13.end
  constraint coincident L4.start L12.start
  constraint coincident L9.end L10.start
  constraint coincident L2.end L3.start
  constraint midpoint L13.end L16
extrude "Extrude4" cut sketch "Sketch4" along normal blind 14 contours L12 L13 L14 L15 L17 L18 L19 L20 L24 | L15 L17 L19 L21 L22 L23 L24 | A1 A2
ref_plane "WorkPlane1" through (9.4113, 3.85, 28.5317) normal (-0.487666, 0, 0.87303) x (0.87303, 0, 0.487666)
sketch "Sketch5" plane through (-9.9091, 0, 17.7395) normal (-0.487666, 0, 0.87303) x (0.87303, 0, 0.487666)
  line L0 (18.9587, 0) -> (11.3502, 0) construction
  line L1 (11.3502, 7.7) -> (18.9587, 7.7) construction
  line L2 (18.9587, 7.7) -> (35.4044, 7.7) construction
  line L3 (35.4044, 7.7) -> (35.4044, 0) construction
  line L4 (35.4044, 0) -> (18.9587, 0) construction
  line L5 (11.3502, 0) -> (27.1815, 0)
  line L6 (27.1815, 0) -> (27.1815, 7.7)
  line L7 (27.1815, 7.7) -> (11.3502, 7.7)
  line L8 (11.3502, 7.7) -> (11.3502, 0)
  line L9 (18.9587, 7.7) -> (18.9587, 0)
  line L10 (11.3502, 0) -> (11.3502, 7.7)
  line L11 (18.9587, 0) -> (18.9587, 7.7)
  circle A0 centre (21.8443, 3.85) radius 2.25
  point P0 (27.1815, 7.7)
  constraint horizontal L5
  constraint vertical L6
  constraint horizontal L7
  constraint vertical L8
  constraint coincident L2 P0
  constraint coincident L0.end L5.start
  constraint midpoint L2 P0
  constraint coincident L6 P0
extrude "Extrude5" cut sketch "Sketch5" against normal blind 15.688 contours L5 L7 L8 L9 L10 L11 | L5 L6 L7 L9 L11 | A0
equation "d19 = d4"
equation "d22 = d1 + 6 mm"

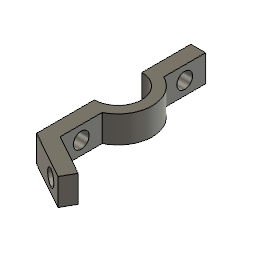
design "Trumpet Clamp 1 Secondary"
Autodesk Fusion 360 part; units mm, degrees
sketch "Sketch1" plane through (0, 0, 0) normal (0, 1, 0) x (1, 0, 0)
  circle A0 centre (0, 0) radius 6.755
  circle A1 centre (0, 0) radius 9.755
  line L0 (0, 0) -> (-9.755, 0) construction
  line L1 (0, 0) -> (9.755, 0) construction
  line L2 (-4.25, -25.7687) -> (18.9274, -38.7154)
  line L3 (4.25, -20.7805) -> (23.0726, -31.2946)
  circle A2 centre (21, -35.005) radius 4.25
  line L4 (21, -35.005) -> (18.9274, -38.7154) construction
  line L5 (21, -35.005) -> (23.0726, -31.2946) construction
  circle A3 centre (21, -35.005) radius 2.25
  line L6 (-4.25, -25.7687) -> (-4.25, -8.7805)
  line L7 (4.25, -20.7805) -> (4.25, -8.7805)
  line L8 (0, 0) -> (0, -20.7805) construction
  line L9 (4.25, -20.7805) -> (-4.25, -20.7805) construction
  line L10 (-4.25, 8.7805) -> (-4.25, 20.7805)
  line L11 (-4.25, 20.7805) -> (4.25, 20.7805)
  line L12 (4.25, 20.7805) -> (4.25, 8.7805)
  line L13 (-4.25, -8.7805) -> (-4.25, 8.7805) construction
  line L14 (4.25, 8.7805) -> (4.25, -8.7805) construction
  line L15 (21, -35.005) -> (21, -39.255) construction
  point P0 (0, -9.755)
  point P1 (21, -39.255)
  dimension "d1" = 13.51
  dimension "d3" = 4.5
  dimension "d4" = 8.5
  dimension "d5" = 21
  dimension "d19" = 8.5
  dimension "d22" = 19.51
  dimension "d31" = 12
  dimension "d32" = 12
  dimension "d35" = 29.5
  constraint coincident A0.centre A1.centre
  constraint concentric A0 A1
  constraint coincident A1 L0.end
  constraint horizontal L0
  constraint coincident A1 L1.end
  constraint parallel L0 L1
  constraint coincident A2.centre L4.start
  constraint coincident A2 L2.end
  constraint coincident A2 L3.end
  constraint parallel L4 L5
  constraint coincident L2.end L4.end
  constraint coincident L3.end L5.end
  constraint coincident A1 L6.end
  constraint coincident A1 L7.end
  constraint parallel L2 L3
  constraint vertical L6
  constraint vertical L7
  constraint vertical L8
  constraint tangent L3 A2
  constraint coincident L6 L9.end
  constraint perpendicular L6 L9
  constraint midpoint L8.end L9
  constraint coincident A1 L10.start
  constraint vertical L10
  constraint perpendicular L10 L11
  constraint coincident A1 L12.end
  constraint perpendicular L11 L12
  constraint vertical L13
  constraint vertical L14
  constraint coincident L8 P0
  constraint coincident A1 P0
  constraint coincident A2 P1
  constraint vertical L15
  constraint coincident P1 L15.end
  measures "d1" diameter of A0
  measures "d3" diameter of A3
  measures "d4" diameter of A2
  measures "d5" horizontal distance of A0.centre A2.centre
  measures "d19" distance of L6 L7
  measures "d22" diameter of A1
  measures "d31" distance of L11.end L12.end
  measures "d32" distance of L3.start L7.end
  measures "d35" vertical distance of P0 P1
extrude "Extrude1" add sketch "Sketch1" along normal blind 7.7
sketch "Sketch2" plane through (-7.8365, 0, 14.0291) normal (0.487666, 0, -0.87303) x (-0.87303, 0, -0.487666)
  line L0 (-35.4044, 0) -> (-13.8443, 0)
  line L1 (-13.8443, 0) -> (-13.8443, 7.7)
  line L2 (-13.8443, 7.7) -> (-35.4044, 7.7)
  line L3 (-35.4044, 7.7) -> (-35.4044, 0)
  line L4 (-13.8443, 3.85) -> (-35.4044, 3.85) construction
  circle A0 centre (-21.8443, 3.85) radius 2.25
  dimension "d33" = 8
  dimension "d34" = 4.5
  constraint midpoint L1 L4.start
  constraint midpoint L3 L4.end
  constraint coincident L4 A0.centre
  measures "d33" distance of L1 A0.centre
  measures "d34" diameter of A0
extrude "Extrude2" cut sketch "Sketch2" against normal up to surface (8.5 mm away) contours A0
sketch "Sketch3" plane through (4.25, 0, 0) normal (1, 0, 0) x (0, 0, -1)
  line L0 (-20.7805, 0) -> (-8.7805, 0)
  line L1 (-8.7805, 0) -> (-8.7805, 7.7)
  line L2 (-8.7805, 7.7) -> (-20.7805, 7.7)
  line L3 (-20.7805, 7.7) -> (-20.7805, 0)
  line L4 (-8.7805, 3.85) -> (-20.7805, 3.85) construction
  circle A0 centre (-14.7805, 3.85) radius 2.25
  line L5 (8.7805, 0) -> (20.7805, 0) construction
  line L6 (20.7805, 0) -> (20.7805, 7.7) construction
  line L7 (20.7805, 7.7) -> (8.7805, 7.7) construction
  line L8 (8.7805, 7.7) -> (8.7805, 0) construction
  line L9 (8.7805, 3.85) -> (20.7805, 3.85) construction
  circle A1 centre (14.7805, 3.85) radius 2.25
  dimension "d16" = 4.5
  constraint midpoint L1 L4.start
  constraint midpoint L3 L4.end
  constraint midpoint L4 A0.centre
  constraint midpoint L8 L9.start
  constraint midpoint L6 L9.end
  constraint midpoint L9 A1.centre
  constraint equal A0 A1
  measures "d16" diameter of A0
extrude "Extrude3" cut sketch "Sketch3" against normal up to surface (8.5 mm away) contours A0 | A1